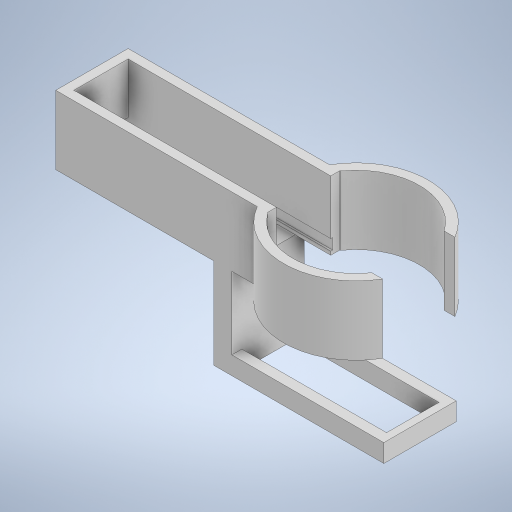
# Autodesk Inventor part: Hovedmagasin
Saved by Autodesk Inventor 2023 (Build 270158000, 158)
## iProperties
Created: 2023-04-11
Part Number: Hovedmagasin
Material: Generic
Document SubType Name: Modeling
Designer: Anders
Density: 1 g/cm^3
Appearance: Default
Author: Anders
## iProperties of the stored document Magasin_3DPrint.ipt
Created: 2023-04-12
Part Number: Magasin_3DPrint
Material: Generic
Document SubType Name: Modeling
Designer: Anders
Density: 1 g/cm^3
Appearance: Default
Author: Anders
Autodesk Inventor part; units mm, degrees
ref_plane "YZ Plane" through (0, 0, 0) normal (1, 0, 0) x (0, 1, 0)
ref_plane "XZ Plane" through (0, 0, 0) normal (0, 1, 0) x (-1, 0, 0)
ref_plane "XY Plane" through (0, 0, 0) normal (0, 0, 1) x (1, 0, 0)
sketch "Sketch1" plane through (0, 0, 0) normal (0, 1, 0) x (-1, 0, 0)
  line L0 (0, 0) -> (60, 0)
  line L1 (60, 0) -> (60, -20)
  line L2 (60, -20) -> (0, -20)
  line L3 (0, -20) -> (0, 0)
  dimension "d0" = 60
  dimension "d1" = 20
  constraints: 8 end point, 2 parallel, 1 horizontal, 1 perpendicular
  measures "d0" distance of L1.end L2.end
  measures "d1" distance of L0.end L1.end
extrude "Extrusion1" add sketch "Sketch1" along normal blind 5
sketch "Sketch2" plane through (0, 5, 0) normal (0, 1, 0) x (1, 0, 0)
  line L0 (0, 20) -> (-60, 20) projected
  line L1 (0, 0) -> (0, 20) projected
  line L2 (-60, 20) -> (0, 20)
  line L3 (0, 20) -> (0, 17.5)
  line L4 (0, 17.5) -> (-60, 17.5)
  line L5 (-60, 17.5) -> (-60, 20)
  line L6 (-60, 20) -> (-60, 0) projected
  line L7 (-60, 0) -> (0, 0)
  line L8 (0, 0) -> (0, 2.5)
  line L9 (0, 2.5) -> (-60, 2.5)
  line L10 (-60, 2.5) -> (-60, 0)
  line L11 (-60, 0) -> (0, 0) projected
  line L12 (-60, 20) -> (-57.5, 20)
  line L13 (-57.5, 20) -> (-57.5, 0)
  line L14 (-57.5, 0) -> (-60, 0)
  line L15 (-60, 0) -> (-60, 20)
  line L16 (0, 20) -> (-2, 20)
  line L17 (-2, 20) -> (-2, 17.5)
  line L18 (-2, 17.5) -> (0, 17.5)
  line L19 (0, 17.5) -> (0, 20)
  line L20 (0, 2.5) -> (-2, 2.5)
  line L21 (-2, 2.5) -> (-2, 0)
  line L22 (-2, 0) -> (0, 0)
  line L23 (0, 0) -> (0, 2.5)
  point P0 (0, 2.5)
  point P1 (-57.5, 2.5)
  point P2 (-57.5, 17.5)
  dimension "d4" = 2.5
  dimension "d5" = 2.5
  dimension "d6" = 2.5
  dimension "d9" = 15
  dimension "d20" = 2
  constraints: 40 end point, 10 parallel, 6 point on line, 5 horizontal, 5 perpendicular
  measures "d4" distance of L2.end L3.end
  measures "d5" distance of L8.end L7.end
  measures "d6" distance of L13.end L14.end
  measures "d9" distance between parallel lines of L4 L9
  measures "d20" distance of L18.end L17.end
extrude "Extrusion2" add sketch "Sketch2" along normal blind 14 contours L1 L4 L17 L0 | L17 L4 L13 L0 | L13 L4 L5 L0 | L1 L7 L21 L9 | L13 L9 L6 L4 | L21 L7 L13 L9 | L13 L7 L6 L9
sketch "Sketch3" plane through (0, 5, 0) normal (0, 1, 0) x (1, 0, 0)
  line L0 (0, 0) -> (0, 2.5) projected
  line L1 (0, 0) -> (26, 0)
  line L2 (26, 0) -> (26, 20)
  line L3 (26, 20) -> (0, 20)
  line L4 (0, 20) -> (0, 0)
  circle A0 centre (13, 10) radius 17.5
  circle A1 centre (13, 10) radius 20
  line L5 (0, 2.5) -> (-57.5, 2.5) projected
  line L6 (0, 2.5) -> (26, 2.5)
  line L7 (26, 2.5) -> (26, 17.5)
  line L8 (26, 17.5) -> (0, 17.5)
  line L9 (0, 17.5) -> (0, 2.5)
  line L10 (0, 17.5) -> (-57.5, 17.5) projected
  line L11 (-57.5, 17.5) -> (-57.5, 2.5) projected
  line L12 (-57.5, 2.5) -> (0, 2.5) projected
  line L13 (0, 2.5) -> (0, 17.5) projected
  line L14 (-5.5405, 2.5) -> (0, 2.5)
  line L15 (-60, 0) -> (0, 0) projected
  line L16 (0, 0) -> (0, 2.5) projected
  line L17 (0, 2.5) -> (-57.5, 2.5) projected
  line L18 (-57.5, 2.5) -> (-57.5, 17.5) projected
  line L19 (-57.5, 17.5) -> (0, 17.5) projected
  line L20 (0, 17.5) -> (0, 20) projected
  line L21 (0, 20) -> (-60, 20) projected
  line L22 (-60, 20) -> (-60, 0) projected
  line L23 (-5.5405, 17.5) -> (0, 17.5)
  line L24 (26, 17.5) -> (31.5405, 17.5)
  line L25 (26, 2.5) -> (31.5405, 2.5)
  line L26 (26, 20) -> (30.3205, 20)
  line L27 (26, 0) -> (30.3205, 0)
  point P0 (-4.3205, 20)
  point P1 (-1.3614, 20)
  point P2 (-1.3614, 0)
  point P3 (-4.3205, 0)
  point P4 (28.8114, 2.5)
  point P5 (28.8114, 17.5)
  point P6 (27.3614, 20)
  point P7 (27.3614, 0)
  dimension "d10" = 26
  dimension "d11" = 20
  dimension "d13" = 35
  dimension "d14" = 40
  dimension "d17" = 15
  constraints: 28 end point, 6 parallel, 6 point on circle, 4 perpendicular, 3 horizontal, 3 point on line, 2 centre point, 1 coincident, 1 collinear
  measures "d10" distance of L3.end L2.end
  measures "d11" distance of L2.end L1.end
  measures "d13" diameter of A0
  measures "d14" diameter of A1
  measures "d17" distance of L7.end L6.end
extrude "Extrusion3" add sketch "Sketch3" along normal blind 14 and the other way blind 5 contours A0 L27 A1 L15 | L21 A1 L26 A0
sketch "Sketch4" plane through (0, 0, 0) normal (0, -1, 0) x (1, 0, 0)
  point P0 (0, 0)
sketch "Sketch5" plane through (0, 0, 0) normal (1, 0, 0) x (0, 0, -1)
  line L0 (17.5, 19) -> (20, 19) projected
  line L1 (0, 0) -> (20, 0) projected
  line L2 (20, 19) -> (17.5, 19)
  line L3 (17.5, 19) -> (17.5, 0)
  line L4 (17.5, 0) -> (20, 0)
  line L5 (20, 0) -> (20, 19)
  line L6 (2.5, 5) -> (2.5, 19) projected
  line L7 (2.5, 19) -> (0, 19)
  line L8 (0, 19) -> (0, 0)
  line L9 (0, 0) -> (2.5, 0)
  line L10 (2.5, 0) -> (2.5, 19)
  line L11 (17.5, 5) -> (2.5, 5)
  line L12 (2.5, 5) -> (2.5, 0)
  line L13 (2.5, 0) -> (17.5, 0)
  line L14 (17.5, 0) -> (17.5, 5)
  dimension "d21" = 2.5
  constraints: 24 end point, 6 parallel, 3 horizontal, 3 perpendicular, 2 point on line
  measures "d21" distance of L4.end L3.end
extrude "Extrusion4" cut sketch "Sketch5" against normal blind 1.5
sketch "Sketch7" plane through (-60, 0, 0) normal (0, 0, 1) x (1, 0, 0)
  line L0 (0, 0) -> (55.6795, 0) projected
  line L1 (55.6795, 0) -> (90.3205, 0) projected
  line L2 (55.6795, 0) -> (55.6795, 19) projected
  line L3 (55.6795, 0) -> (48.6795, 0)
  line L4 (48.6795, 0) -> (48.6795, -25)
  line L5 (48.6795, -25) -> (55.6795, -25)
  line L6 (55.6795, -25) -> (55.6795, 0)
  line L7 (55.6795, -25) -> (90.6795, -25)
  line L8 (90.6795, -25) -> (90.6795, -20)
  line L9 (90.6795, -20) -> (55.6795, -20)
  line L10 (55.6795, -20) -> (55.6795, -25)
  point P0 (60, 0)
  dimension "d25" = 7
  dimension "d26" = 25
  dimension "d27" = 35
  dimension "d28" = 5
  constraints: 16 end point, 4 parallel, 2 horizontal, 2 perpendicular
  measures "d25" distance of L5.end L4.end
  measures "d26" distance of L4.end L3.end
  measures "d27" distance of L9.end L8.end
  measures "d28" distance of L8.end L7.end
extrude "Extrusion5" add sketch "Sketch7" against normal up to surface (20 mm away)
sketch "Sketch8" plane through (0, 0, 0) normal (0, -1, 0) x (1, 0, 0)
  point P0 (0, 0)
sketch "Sketch9" plane through (-11.3205, -25, 0) normal (0, -1, 0) x (1, 0, 0)
  line L0 (0, -20) -> (42, -20) projected
  line L1 (0, 0) -> (42, 0) projected
  arc A0 (7, -20) -> (41.641, -20) centre (24.3205, -10) ccw projected
  line L2 (42.861, -17.5) -> (40.1319, -17.5) projected
  arc A1 (9.9591, -20) -> (38.6819, -20) centre (24.3205, -10) ccw projected
  line L3 (9.9591, -20) -> (9.8205, -20) projected
  line L4 (9.8205, 0) -> (9.9591, 0) projected
  arc A2 (38.6819, 0) -> (9.9591, 0) centre (24.3205, -10) ccw projected
  line L5 (40.1319, -2.5) -> (42.861, -2.5) projected
  arc A3 (41.641, 0) -> (7, 0) centre (24.3205, -10) ccw projected
  line L6 (5, -2.75) -> (40, -2.75)
  line L7 (40, -2.75) -> (40, -17.25)
  line L8 (40, -17.25) -> (5, -17.25)
  line L9 (5, -17.25) -> (5, -2.75)
  line L10 (0, 0) -> (0, -20) projected
  point P0 (11.3205, 0)
  point P1 (5, -10)
  dimension "d36" = 35
  dimension "d37" = 14.5
  dimension "d38" = 5
  dimension "d39" = 2.75
  constraints: 8 end point, 4 centre point, 2 parallel, 1 horizontal, 1 midpoint, 1 perpendicular
  measures "d36" distance of L7.end L8.end
  measures "d37" distance of L6.end L7.end
  measures "d38" distance from line of point (5, -10) L10
  measures "d39" distance between parallel lines of L1 L6
extrude "Extrusion6" cut sketch "Sketch9" against normal blind 10 contours L6 L7 L8 L9
sketch "Sketch10" plane through (-1.5, 0, 0) normal (1, 0, 0) x (0, 0, -1)
  line L0 (2.5, 5) -> (17.5, 5) projected
  line L1 (2.5, 19) -> (2.5, 5) projected
  line L2 (17.5, 5) -> (17.5, 19) projected
  line L3 (20, 0) -> (0, 0) projected
  line L4 (2.5, 5) -> (17.5, 5)
  line L5 (17.5, 5) -> (17.5, 0)
  line L6 (17.5, 0) -> (2.5, 0)
  line L7 (2.5, 0) -> (2.5, 5)
  line L8 (2.5, 4) -> (2, 4)
  line L9 (2, 4) -> (2, 1)
  line L10 (2, 1) -> (2.5, 1)
  line L11 (2.5, 1) -> (2.5, 4)
  line L12 (0, 0) -> (0, 19) projected
  line L13 (17.5, 4) -> (18, 4)
  line L14 (18, 4) -> (18, 1)
  line L15 (18, 1) -> (17.5, 1)
  line L16 (17.5, 1) -> (17.5, 4)
  line L17 (20, 19) -> (20, 0) projected
  point P0 (2.25, 4)
  point P1 (2.25, 1)
  point P2 (18, 2.5)
  point P3 (17.75, 1)
  point P4 (17.75, 4)
  point P5 (17.5, 1)
  point P6 (2.5, 1)
  dimension "d42" = 2
  dimension "d43" = 1
  dimension "d44" = 1
  dimension "d45" = 2
  dimension "d46" = 1
  dimension "d47" = 1
  dimension "d49" = 2.5
  constraints: 24 end point, 6 parallel, 5 midpoint, 3 horizontal, 3 perpendicular, 3 point on line
  measures "d42" distance between parallel lines of L12 L9
  measures "d43" distance from line of L0 point (2.25, 4)
  measures "d44" distance from line of L3 point (2.25, 1)
  measures "d45" distance from line of L17 point (18, 2.5)
  measures "d46" distance from line of L3 point (17.75, 1)
  measures "d47" distance from line of L0 point (17.75, 4)
  measures "d49" distance between parallel lines of L17 L16
extrude "Extrusion7" cut sketch "Sketch10" against normal through all
sketch "Sketch11" plane through (-11.3205, -25, 0) normal (-1, 0, 0) x (0, 0, 1)
  line L0 (0, 25) -> (0, 0) projected
  line L1 (-20, 25) -> (-20, 0) projected
  line L2 (0, 0) -> (-20, 0)
  line L3 (-20, 0) -> (-20, 25)
  line L4 (-20, 25) -> (0, 25)
  line L5 (0, 25) -> (0, 0)
  constraints: 8 end point, 2 parallel, 1 horizontal, 1 perpendicular
extrude "Extrusion8" add sketch "Sketch11" along normal blind 5
sketch "Sketch12" plane through (-4.3205, -20, 0) normal (1, 0, 0) x (0, 0, -1)
  line L0 (2.75, 5) -> (17.25, 5) projected
  line L1 (17.25, 0) -> (20, 0) projected
  line L2 (17.25, 5) -> (20, 5)
  line L3 (20, 5) -> (20, 0)
  line L4 (20, 0) -> (17.25, 0)
  line L5 (17.25, 0) -> (17.25, 5)
  line L6 (2.75, -5) -> (2.75, 5) projected
  line L7 (0, -5) -> (0, 20) projected
  line L8 (2.75, 5) -> (0, 5)
  line L9 (0, 5) -> (0, 0)
  line L10 (0, 0) -> (2.75, 0)
  line L11 (2.75, 0) -> (2.75, 5)
  line L12 (0, 20) -> (2.5, 20) projected
  line L13 (20, 5) -> (0, 5)
  line L14 (0, 5) -> (0, 20)
  line L15 (0, 20) -> (20, 20)
  line L16 (20, 20) -> (20, 5)
  point P0 (2.75, 0)
  constraints: 24 end point, 6 parallel, 3 horizontal, 3 perpendicular, 2 point on line
extrude "Extrusion9" cut sketch "Sketch12" against normal blind 7
sketch "Sketch13" plane through (-6.3205, -25, -2.75) normal (1, 0, 0) x (0, 0, -1)
  line L0 (0, 0) -> (0, 5) projected
  line L1 (14.5, 10) -> (0, 10)
  line L2 (0, 10) -> (0, 0)
  line L3 (0, 0) -> (14.5, 0)
  line L4 (14.5, 0) -> (14.5, 10)
  point P0 (-2.75, 25)
  point P1 (0, 5)
  constraints: 8 end point, 2 parallel, 1 horizontal, 1 perpendicular
extrude "Extrusion10" cut sketch "Sketch13" against normal blind 5
sketch "Sketch14" plane through (-1.5, 19, -2.5) normal (0, 0, -1) x (-1, 0, 0)
  point P0 (-1.5, -19)
body "Solid1"
